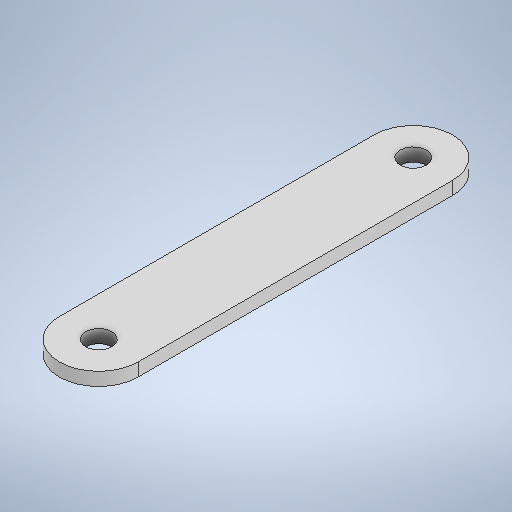
# Autodesk Inventor part: Coupler Link
Saved by Autodesk Inventor 2025 (Build 290162000, 162)
## iProperties
Created: 2025-11-15
Part Number: Coupler Link
Material: Generic
Document SubType Name: Modeling
Designer: parsh
Density: 1 g/cm^3
Appearance: Default
Author: parsh
Autodesk Inventor part; units mm, degrees
ref_plane "YZ Plane" through (0, 0, 0) normal (1, 0, 0) x (0, 1, 0)
ref_plane "XZ Plane" through (0, 0, 0) normal (0, 1, 0) x (-1, 0, 0)
ref_plane "XY Plane" through (0, 0, 0) normal (0, 0, 1) x (1, 0, 0)
sketch "Sketch1" plane through (0, 0, 0) normal (0, 1, 0) x (-1, 0, 0)
  line L0 (0, 0) -> (30, 0)
  line L1 (30, 0) -> (30, -150)
  line L2 (30, -150) -> (0, -150)
  line L3 (0, -150) -> (0, 0)
  dimension "d0" = 30
  dimension "d1" = 150
  constraints: 8 end point, 2 parallel, 1 horizontal, 1 perpendicular
  measures "d0" distance of L1.end L2.end
  measures "d1" distance of L0.end L1.end
extrude "Extrusion1" add sketch "Sketch1" along normal blind 5
fillet "Fillet1" radius 15 4 edges at (0, 2.5, 0) (-30, 2.5, 0) (0, 2.5, -150) (-30, 2.5, -150)
sketch "Sketch2" plane through (0, 5, 0) normal (0, 1, 0) x (1, 0, 0)
  arc A0 (0, 135) -> (-30, 135) centre (-15, 135) ccw projected
  circle A1 centre (-15, 135) radius 5
  arc A2 (-30, 15) -> (0, 15) centre (-15, 15) ccw projected
  circle A3 centre (-15, 15) radius 5
  point P0 (0, 0)
  dimension "d5" = 10
  dimension "d6" = 10
  constraints: 2 centre point, 2 coincident
  measures "d5" diameter of A1
  measures "d6" diameter of A3
extrude "Extrusion2" cut sketch "Sketch2" against normal blind 10
equation "\"d7\" = d6"
body "Solid1"
